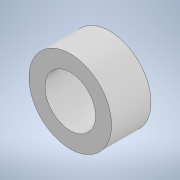
# Autodesk Inventor part: threadSpacer
Saved by Autodesk Inventor 2020 (Build 240168000, 168)
## iProperties
Created: 2019-10-16
Part Number: threadSpacer
Material: Generic
Document SubType Name: Modeling
Designer: Acer
Density: 1 g/cm^3
Appearance: Default
Author: Acer
Autodesk Inventor part; units mm, degrees
ref_plane "YZ Plane" through (0, 0, 0) normal (1, 0, 0) x (0, 1, 0)
ref_plane "XZ Plane" through (0, 0, 0) normal (0, 1, 0) x (-1, 0, 0)
ref_plane "XY Plane" through (0, 0, 0) normal (0, 0, 1) x (1, 0, 0)
sketch "Sketch1" plane through (0, 0, 0) normal (0, 0, 1) x (1, 0, 0)
  circle A0 centre (0, 0) radius 4.975
  circle A1 centre (0, 0) radius 3.05
  dimension "d0" = 9.95
  dimension "d1" = 6.1
  constraints: 2 centre point, 2 coincident
  measures "d0" diameter of A0
  measures "d1" diameter of A1
extrude "Extrusion1" add sketch "Sketch1" along normal blind 4.75
body "Solid1"
